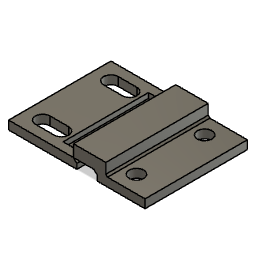
Curtain Clamps Side slide v4 (Autodesk Fusion 360 design; units mm, degrees)
Autodesk Fusion 360 part; units mm, degrees
sketch "Sketch1" plane through (0, 0, 0) normal (0, 1, 0) x (1, 0, 0)
  line L0 (20, 30) -> (-20, 30)
  line L1 (-20, 30) -> (-20, -30)
  line L2 (-20, -30) -> (20, -30)
  line L3 (20, -30) -> (20, 30)
  line L4 (20, 30) -> (-20, -30) construction
  line L5 (-20, 30) -> (20, -30) construction
  circle A0 centre (-10, 20) radius 4.25
  circle A1 centre (1, 20) radius 4.25
  circle A2 centre (-10, -20) radius 4.25
  circle A3 centre (1, -20) radius 4.25
  line L6 (-10, 15.75) -> (1, 15.75)
  line L7 (1, 15.75) -> (1, 24.25)
  line L8 (1, 24.25) -> (-10, 24.25)
  line L9 (-10, 24.25) -> (-10, 15.75)
  line L10 (-10, -24.25) -> (1, -24.25)
  line L11 (1, -24.25) -> (1, -15.75)
  line L12 (1, -15.75) -> (-10, -15.75)
  line L13 (-10, -15.75) -> (-10, -24.25)
  dimension "d1" = 40
  dimension "d2" = 60
  dimension "d3" = 8.5
  dimension "d4" = 8.5
  dimension "d5" = 8.5
  dimension "d6" = 8.5
  constraint horizontal L0
  constraint perpendicular L0 L1
  constraint parallel L0 L2
  constraint parallel L1 L3
  constraint coincident L4 origin
  constraint coincident L5 origin
  constraint perpendicular L6 L7
  constraint parallel L6 L8
  constraint parallel L7 L9
  constraint coincident A1 L6.end
  constraint tangent A1 L6
  constraint horizontal L6
  constraint coincident A0 L6.start
  constraint perpendicular L10 L11
  constraint parallel L10 L12
  constraint parallel L11 L13
  constraint coincident A3 L10.end
  constraint tangent A3 L10
  constraint perpendicular L9 L10
  constraint coincident A2 L10.start
  measures "d1" distance of L1.end L2.end
  measures "d2" distance of L0.end L1.end
  measures "d3" diameter of A0
  measures "d4" diameter of A1
  measures "d5" diameter of A2
  measures "d6" diameter of A3
extrude "Extrude1" add sketch "Sketch1" along normal blind 5 makes body 1
sketch "Sketch4" plane through (0, 0, 0) normal (0, 1, 0) x (1, 0, 0)
  line L0 (30, 30) -> (60, 30)
  line L1 (60, 30) -> (60, -30)
  line L2 (60, -30) -> (30, -30)
  line L3 (30, -30) -> (30, 30)
  circle A0 centre (45, 20) radius 4.25
  circle A1 centre (45, -20) radius 4.25
  dimension "d18" = 8.5
  dimension "d19" = 8.5
  constraint horizontal L0
  constraint vertical L1
  constraint horizontal L2
  constraint vertical L3
  measures "d18" diameter of A0
  measures "d19" diameter of A1
extrude "Extrude4" add sketch "Sketch4" along normal blind 5 separate body makes body 2
sketch "Sketch6" plane through (0, 5, 0) normal (0, 1, 0) x (-1, 0, 0)
  circle A0 centre (-45, -20) radius 4.25
  circle A1 centre (-45, 20) radius 4.25
  line L0 (-30, 30) -> (-60, 30)
  line L1 (-60, 30) -> (-60, -30)
  line L2 (-60, -30) -> (-30, -30)
  line L3 (-30, -30) -> (-30, 30)
  line L4 (-30, -30) -> (-37, -30)
  line L5 (-37, -30) -> (-37, 30)
  line L6 (-37, 30) -> (-30, 30)
  line L7 (-30, 30) -> (-30, -30)
  constraint horizontal L4
  constraint vertical L5
  constraint horizontal L6
  constraint vertical L7
  constraint coincident L0 L5.end
  constraint coincident L2.end L3.start
extrude "Extrude7" add sketch "Sketch6" along normal blind 7 contours L0 L2 L3 L4 L5 L6 L7 bodies 2
sketch "Sketch7" plane through (30, 0, 0) normal (-1, 0, 0) x (0, 0, 1)
  line L0 (-30, 0) -> (30, 0)
  line L1 (30, 0) -> (30, 12)
  line L2 (30, 12) -> (-30, 12)
  line L3 (-30, 12) -> (-30, 0)
  line L4 (-30, 12) -> (30, 12)
  line L5 (30, 12) -> (30, 5)
  line L6 (30, 5) -> (-30, 5)
  line L7 (-30, 5) -> (-30, 12)
  constraint horizontal L4
  constraint vertical L5
  constraint horizontal L6
  constraint vertical L7
  constraint coincident L1 L5.end
  constraint coincident L2.end L3.start
extrude "Extrude9" add sketch "Sketch7" along normal blind 12 contours L1 L2 L3 L4 L5 L6 L7 bodies 2
sketch "Sketch8" plane through (0, 5, 0) normal (0, 1, 0) x (-1, 0, 0)
  line L0 (10, 15.75) -> (-1, 15.75)
  arc A0 (-1, 24.25) -> (-1, 15.75) centre (-1, 20) ccw
  line L1 (-1, 24.25) -> (10, 24.25)
  arc A1 (10, 15.75) -> (10, 24.25) centre (10, 20) ccw
  line L2 (10, -24.25) -> (-1, -24.25)
  arc A2 (-1, -15.75) -> (-1, -24.25) centre (-1, -20) ccw
  line L3 (-1, -15.75) -> (10, -15.75)
  arc A3 (10, -24.25) -> (10, -15.75) centre (10, -20) ccw
  line L4 (-20, 30) -> (-20, -30)
  line L5 (-20, -30) -> (20, -30)
  line L6 (20, -30) -> (20, 30)
  line L7 (20, 30) -> (-20, 30)
  line L8 (-7, -25) -> (-17, -25)
  line L9 (-17, -25) -> (-17, 25)
  line L10 (-17, 25) -> (-7, 25)
  line L11 (-7, 25) -> (-7, -25)
  constraint horizontal L8
  constraint vertical L9
  constraint horizontal L10
  constraint vertical L11
extrude "Extrude10" cut sketch "Sketch8" against normal blind 3 contours L8 L9 L10 L11 bodies 1
sketch "Sketch9" plane through (0, 5, 0) normal (0, -1, 0) x (1, 0, 0)
  line L0 (30, -30) -> (30, 30)
  line L1 (30, 30) -> (18, 30)
  line L2 (18, 30) -> (18, -30)
  line L3 (18, -30) -> (30, -30)
  circle A0 centre (24, 20) radius 3
  circle A1 centre (24, 0) radius 3
  circle A2 centre (24, -20) radius 3
extrude "Extrude11" cut sketch "Sketch9" against normal blind 4 contours A0 | A1 | A2 bodies 2
extrude "Extrude12" cut 1 faces at (30, 1.6667, 10) along direction (1, 0, 0) blind 2 on bodies 2 bodies 2
chamfer "Chamfer1" distance 2 angle 45 1 edges at (20, 5, 0) on bodies 1
chamfer "Chamfer2" distance 2 angle 45 1 edges at (32, 5, 0) on bodies 2
chamfer "Chamfer3" distance 1 angle 45 1 edges at (37, 5, 0) on bodies 2
